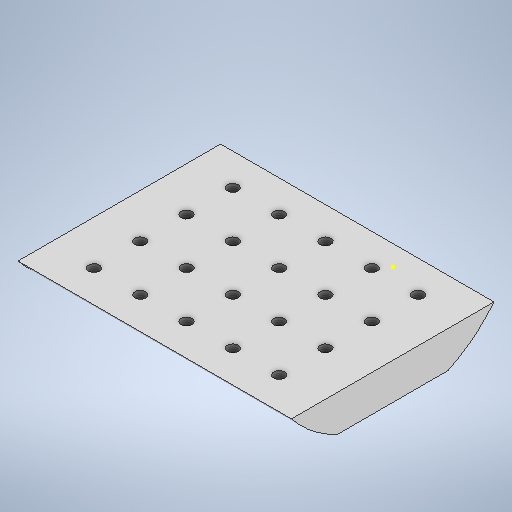
# Autodesk Inventor part: Base
Saved by Autodesk Inventor 2025.3 (Build 293356000, 356)
## iProperties
Created: 2025-05-16
Part Number: Base
Material: Generic
Document SubType Name: Modeling
Designer: Verðandi
Density: 1 g/cm^3
Appearance: Default
Author: Verðandi
Autodesk Inventor part; units mm, degrees
ref_plane "YZ Plane" through (0, 0, 0) normal (1, 0, 0) x (0, 1, 0)
ref_plane "XZ Plane" through (0, 0, 0) normal (0, 1, 0) x (-1, 0, 0)
ref_plane "XY Plane" through (0, 0, 0) normal (0, 0, 1) x (1, 0, 0)
sketch "Sketch1" plane through (0, 0, 0) normal (1, 0, 0) x (0, 1, 0)
  circle A0 centre (0, 0) radius 71
  dimension "d0" = 142
  constraints: 1 centre point, 1 coincident
  measures "d0" diameter of A0
extrude "Extrusion1" add sketch "Sketch1" along normal blind 150
sketch "Sketch2" plane through (150, 0, 0) normal (1, 0, 0) x (0, 0, -1)
  line L0 (0, 0) -> (0, -44.2)
  circle A0 centre (0, 0) radius 71 projected
  line L1 (-55.564, -44.2) -> (55.564, -44.2)
  dimension "d3" = 44.2
  constraints: 4 end point, 2 point on circle, 1 horizontal, 1 vertical
  measures "d3" distance of L0.start L0.end
extrude "Extrusion2" cut sketch "Sketch2" against normal blind 150 contours A0 L1 picked at (-0.2063, 32.437)
sketch "Sketch3" plane through (150, 0, 0) normal (1, 0, 0) x (0, 0, -1)
  line L0 (0, 0) -> (0, -64.2)
  arc A0 (-55.564, -44.2) -> (55.564, -44.2) centre (0, 0) ccw projected
  line L1 (-30.3209, -64.2) -> (30.3209, -64.2)
  dimension "d6" = 64.2
  constraints: 4 end point, 2 point on circle, 1 horizontal, 1 vertical
  measures "d6" distance of L0.start L0.end
sketch "Sketch5" plane through (150, -44.2, 55.564) normal (0, 1, 0) x (1, 0, 0)
  line L0 (-150, 55.564) -> (-75, 55.564)
  line L1 (-75, 55.564) -> (-75, 68.264)
  line L2 (-75, 55.564) -> (-75, 42.864)
  circle A0 centre (-75, 68.264) radius 3
  circle A1 centre (-75, 42.864) radius 3
  line L3 (-75, 68.264) -> (-49.6, 68.264)
  line L4 (-75, 42.864) -> (-49.6, 42.864)
  line L5 (-75, 68.264) -> (-100.4, 68.264)
  line L6 (-75, 42.864) -> (-100.4, 42.864)
  circle A2 centre (-100.4, 68.264) radius 3
  circle A3 centre (-49.6, 68.264) radius 3
  circle A4 centre (-49.6, 42.864) radius 3
  circle A5 centre (-100.4, 42.864) radius 3
  line L7 (-100.4, 42.864) -> (-125.8, 42.864)
  line L8 (-100.4, 68.264) -> (-125.8, 68.264)
  line L9 (-49.6, 68.264) -> (-24.2, 68.264)
  line L10 (-49.6, 42.864) -> (-24.2, 42.864)
  circle A6 centre (-125.8, 68.264) radius 3
  circle A7 centre (-125.8, 42.864) radius 3
  circle A8 centre (-24.2, 68.264) radius 3
  circle A9 centre (-24.2, 42.864) radius 3
  line L11 (-125.8, 68.264) -> (-125.8, 93.664)
  line L12 (-100.4, 68.264) -> (-100.4, 93.664)
  line L13 (-75, 68.264) -> (-75, 93.664)
  line L14 (-75, 68.264) -> (-49.6, 68.264) construction
  line L15 (-49.6, 68.264) -> (-49.6, 93.664)
  line L16 (-24.2, 68.264) -> (-24.2, 93.664)
  line L17 (-125.8, 42.864) -> (-125.8, 17.464)
  line L18 (-100.4, 42.864) -> (-100.4, 17.464)
  line L19 (-75, 42.864) -> (-75, 17.464)
  line L20 (-49.6, 42.864) -> (-49.6, 17.464)
  line L21 (-24.2, 42.864) -> (-24.2, 17.464)
  circle A10 centre (-125.8, 93.664) radius 3
  circle A11 centre (-100.4, 93.664) radius 3
  circle A12 centre (-75, 93.664) radius 3
  circle A13 centre (-49.6, 93.664) radius 3
  circle A14 centre (-24.2, 93.664) radius 3
  circle A15 centre (-24.2, 17.464) radius 3
  circle A16 centre (-49.6, 17.464) radius 3
  circle A17 centre (-75, 17.464) radius 3
  circle A18 centre (-100.4, 17.464) radius 3
  circle A19 centre (-125.8, 17.464) radius 3
  dimension "d9" = 75
  dimension "d10" = 12.7
  dimension "d11" = 12.7
  dimension "d12" = 6
  dimension "d13" = 6
  dimension "d14" = 25.4
  dimension "d15" = 25.4
  dimension "d16" = 25.4
  dimension "d17" = 25.4
  dimension "d18" = 6
  dimension "d19" = 6
  dimension "d20" = 6
  dimension "d21" = 6
  dimension "d22" = 25.4
  dimension "d23" = 25.4
  dimension "d24" = 25.4
  dimension "d25" = 25.4
  dimension "d26" = 6
  dimension "d27" = 6
  dimension "d28" = 6
  dimension "d29" = 6
  dimension "d30" = 25.4
  dimension "d31" = 25.4
  dimension "d32" = 25.4
  dimension "d33" = 90
  dimension "d34" = 25.4
  dimension "d35" = 25.4
  dimension "d36" = 25.4
  dimension "d37" = 25.4
  dimension "d38" = 25.4
  dimension "d39" = 25.4
  dimension "d40" = 25.4
  dimension "d41" = 6
  dimension "d42" = 6
  dimension "d43" = 6
  dimension "d44" = 6
  dimension "d45" = 6
  dimension "d46" = 6
  dimension "d47" = 6
  dimension "d48" = 6
  dimension "d49" = 6
  dimension "d50" = 6
  constraints: 44 end point, 20 centre point, 20 coincident, 10 horizontal, 10 vertical, 3 perpendicular
  measures "d9" distance of L0.start L0.end
  measures "d10" distance of L0.end L1.end
  measures "d11" distance of L0.end L2.end
  measures "d12" diameter of A0
  measures "d13" diameter of A1
  measures "d14" distance of L3.start L3.end
  measures "d15" distance of L4.start L4.end
  measures "d16" distance of L3.start L5.end
  measures "d17" distance of L4.start L6.end
  measures "d18" diameter of A2
  measures "d19" diameter of A3
  measures "d20" diameter of A4
  measures "d21" diameter of A5
  measures "d22" distance of L7.start L7.end
  measures "d23" distance of L8.start L8.end
  measures "d24" distance of L9.start L9.end
  measures "d25" distance of L10.start L10.end
  measures "d26" diameter of A6
  measures "d27" diameter of A7
  measures "d28" diameter of A8
  measures "d29" diameter of A9
  measures "d30" distance of L11.start L11.end
  measures "d31" distance of L8.start L12.end
  measures "d32" distance of L3.start L13.end
  measures "d33" angle of L14 L13
  measures "d34" distance of L14.end L15.end
  measures "d35" distance of L16.start L16.end
  measures "d36" distance of L17.start L17.end
  measures "d37" distance of L7.start L18.end
  measures "d38" distance of L4.start L19.end
  measures "d39" distance of L10.start L20.end
  measures "d40" distance of L21.start L21.end
  measures "d41" diameter of A10
  measures "d42" diameter of A11
  measures "d43" diameter of A12
  measures "d44" diameter of A13
  measures "d45" diameter of A14
  measures "d46" diameter of A15
  measures "d47" diameter of A16
  measures "d48" diameter of A17
  measures "d49" diameter of A18
  measures "d50" diameter of A19
sketch "Sketch6" plane through (150, 0, 0) normal (1, 0, 0) x (0, 0, -1)
  point P0 (0, 0)
extrude "Extrusion4" cut sketch "Sketch3" against normal blind 150
extrude "Extrusion5" cut sketch "Sketch5" against normal blind 10
thread "Thread1" size "M6x1" class "6H" standard "ANSI Metric M Profile" full length
thread "Thread2" size "M6x1" class "6H" standard "ANSI Metric M Profile" full length
thread "Thread3" size "M6x1" class "6H" standard "ANSI Metric M Profile" full length
thread "Thread4" size "M6x1" class "6H" standard "ANSI Metric M Profile" full length
thread "Thread5" size "M6x1" class "6H" standard "ANSI Metric M Profile" full length
thread "Thread6" size "M6x1" class "6H" standard "ANSI Metric M Profile" full length
thread "Thread7" size "M6x1" class "6H" standard "ANSI Metric M Profile" full length
thread "Thread8" size "M6x1" class "6H" standard "ANSI Metric M Profile" full length
thread "Thread9" size "M6x1" class "6H" standard "ANSI Metric M Profile" full length
thread "Thread10" size "M6x1" class "6H" standard "ANSI Metric M Profile" full length
thread "Thread11" size "M6x1" class "6H" standard "ANSI Metric M Profile" full length
thread "Thread12" size "M6x1" class "6H" standard "ANSI Metric M Profile" full length
thread "Thread13" size "M6x1" class "6H" standard "ANSI Metric M Profile" full length
thread "Thread14" size "M6x1" class "6H" standard "ANSI Metric M Profile" full length
thread "Thread15" size "M6x1" class "6H" standard "ANSI Metric M Profile" full length
thread "Thread16" size "M6x1" class "6H" standard "ANSI Metric M Profile" full length
thread "Thread17" size "M6x1" class "6H" standard "ANSI Metric M Profile" full length
thread "Thread18" size "M6x1" class "6H" standard "ANSI Metric M Profile" full length
thread "Thread19" size "M6x1" class "6H" standard "ANSI Metric M Profile" full length
thread "Thread20" size "M6x1" class "6H" standard "ANSI Metric M Profile" full length
body "Solid1"
